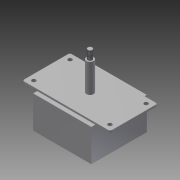
# Autodesk Inventor part: JLF-TP-8YT_body
Saved by Autodesk Inventor 2013 (Build 170138000, 138)
## iProperties
Created: 2013-01-27
Part Number: JLF-TP-8YT_body
Material: Steel AISI 4620
Document SubType Name: Modeling
Designer: xylzlyx
Density: 1 g/cm^3
Author: xylzlyx
Autodesk Inventor part; units mm, degrees
ref_plane "YZ Plane" through (0, 0, 0) normal (1, 0, 0) x (0, 1, 0)
ref_plane "XZ Plane" through (0, 0, 0) normal (0, 1, 0) x (-1, 0, 0)
ref_plane "XY Plane" through (0, 0, 0) normal (0, 0, 1) x (1, 0, 0)
sketch "JoystickMount" plane through (0, 0, 0) normal (0, 0, 1) x (1, 0, 0)
  line L0 (-49, 26.5) -> (49, 26.5)
  line L1 (49, 26.5) -> (49, -26.5)
  line L2 (49, -26.5) -> (-49, -26.5)
  line L3 (-49, -26.5) -> (-49, 26.5)
  point P0 (0, 0)
  point P1 (-49, 0)
  point P2 (0, 26.5)
  point P3 (0, -26.5)
  point P4 (49, 0)
  dimension "d0" = 53
  dimension "d2" = 98
  constraints: 8 end point, 4 midpoint, 2 horizontal alignment, 2 parallel, 2 vertical alignment, 1 horizontal, 1 perpendicular
  measures "d0" distance of L2.end L0.start
  measures "d2" distance of L0.start L0.end
extrude "JoystickMountPlate" add sketch "JoystickMount" against normal blind 2
fillet "MountPlateCornerFillet" radius 2 4 edges at (49, 26.5, -1) (-49, 26.5, -1) (-49, -26.5, -1) (49, -26.5, -1)
sketch "BodySketch" plane through (0, 0, -2) normal (0, 0, -1) x (-1, 0, 0)
  line L0 (-32.5, 31) -> (32.5, 31)
  line L1 (32.5, 31) -> (32.5, -31)
  line L2 (32.5, -31) -> (-32.5, -31)
  line L3 (-32.5, -31) -> (-32.5, 31)
  point P0 (0, 0)
  point P1 (-32.5, 0)
  point P2 (0, 31)
  dimension "d6" = 65
  dimension "d8" = 62
  constraints: 8 end point, 2 midpoint, 2 parallel, 1 horizontal, 1 horizontal alignment, 1 perpendicular, 1 vertical alignment
  measures "d6" distance of L0.start L0.end
  measures "d8" distance of L2.end L0.start
extrude "JoystickBody" add sketch "BodySketch" along normal blind 36
sketch "JoystickPostCenter" plane through (0, 0, 0) normal (0, 0, 1) x (1, 0, 0)
  circle A0 centre (0, 0) radius 4
  dimension "d11" = 8
  constraints: 3 coincident, 1 centre point
  measures "d11" diameter of A0
extrude "Shaft" add sketch "JoystickPostCenter" along normal blind 32
sketch "ThreadSketch" plane through (0, 0, 32) normal (0, 0, 1) x (1, 0, 0)
  circle A0 centre (0, 0) radius 4 projected
  circle A1 centre (0, 0) radius 2.5
  dimension "d14" = 5
  constraints: 1 centre point, 1 coincident
  measures "d14" diameter of A1
extrude "ShaftScrew" add sketch "ThreadSketch" along normal blind 10 contours A1
thread "ShaftThread" size "M5x0.8" class "6g" standard "ANSI Metric M Profile" full length
sketch "MountHoles" plane through (0, 0, 0) normal (0, 0, 1) x (1, 0, 0)
  circle A0 centre (0, 0) radius 4 projected
  line L0 (47, -26.5) -> (-47, -26.5) projected
  line L1 (-42.5, 20.25) -> (-42.5, -20.25) construction
  line L2 (-42.5, -20.25) -> (42.5, -20.25) construction
  point P0 (42.5, 20.25)
  point P1 (-42.5, 0)
  point P2 (0, -20.25)
  dimension "d44" = 40.5
  dimension "d46" = 85
  constraints: 4 end point, 3 horizontal alignment, 3 vertical alignment, 2 midpoint, 2 perpendicular
  measures "d44" distance of L1.end L1.start
  measures "d46" distance of L2.end L1.end
hole "MountingHoles" at (-42.5, 20.25, 0) at (-42.5, -20.25, 0) at (42.5, -20.25, 0) at (42.5, 20.25, 0) direction (0, 0, -1) diameter 4.5 end through all clearance for "Flat Head Machine Screw" size "M4" standard "Ansi Metric M Profile"
body "Solid1"
